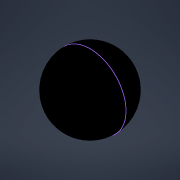
# Autodesk Inventor part: DOME
Saved by Autodesk Inventor 2022 (Build 260153070, 153G)
## iProperties
Created: 2021-11-19
Part Number: DOME
Material: Каучук, черный
Document SubType Name: Modeling
Designer: kalugin_a
Density: 0.93 g/cm^3
Appearance: Оксидированная
Author: kalugin_a
Autodesk Inventor part; units mm, degrees
ref_plane "YZ Plane" through (0, 0, 0) normal (1, 0, 0) x (0, 1, 0)
ref_plane "XZ Plane" through (0, 0, 0) normal (0, 1, 0) x (-1, 0, 0)
ref_plane "XY Plane" through (0, 0, 0) normal (0, 0, 1) x (1, 0, 0)
sketch "Эскиз2" plane through (0, 0, 0) normal (0, 0, 1) x (1, 0, 0)
  circle A0 centre (0, 0) radius 19.159
  line L0 (13.1958, -13.8903) -> (-13.1958, 13.8903)
  dimension "d1" = 360
  constraints: 2 end point, 2 point on circle, 1 centre point, 1 coincident, 1 midpoint
revolve "Вращение2" add sketch "Эскиз2" angle 360 about axis through (13.1958, -13.8903, 0) along (-0.6887495, 0.7249994, 0) picked at (8.4168, 1.8713) contours A0 L0
